Encoder 14bit v5 (Autodesk Fusion 360 design; units mm, degrees)
Autodesk Fusion 360 part; units mm, degrees
sketch "Sketch1" plane through (0, 0, 0) normal (0, 0, 1) x (1, 0, 0)
  circle A0 centre (-8.5, 8.5) radius 1
  line L0 (-10.5, 11.5) -> (10.5, 11.5)
  line L1 (11.5, 10.5) -> (11.5, -10.5)
  line L2 (10.5, -11.5) -> (-10.5, -11.5)
  line L3 (-11.5, -10.5) -> (-11.5, 10.5)
  line L4 (-9.5, 11.5) -> (-9.5, 8.5) construction
  line L5 (-7.5, 11.5) -> (-7.5, 8.5) construction
  line L6 (-8.5, 9.5) -> (-11.5, 9.5) construction
  line L7 (0, 11.5) -> (0, -11.5) construction
  line L8 (-11.5, 0) -> (11.5, 0) construction
  circle A1 centre (8.5, 8.5) radius 1
  circle A2 centre (8.5, -8.5) radius 1
  circle A3 centre (-8.5, -8.5) radius 1
  line L9 (-10.5, 11.5) -> (-11.5, 10.5)
  line L10 (10.5, 11.5) -> (11.5, 10.5)
  line L11 (11.5, -10.5) -> (10.5, -11.5)
  line L12 (-10.5, -11.5) -> (-11.5, -10.5)
  point P0 (-11.5, 11.5)
  point P1 (11.5, 11.5)
  point P2 (11.5, -11.5)
  point P3 (-11.5, -11.5)
  dimension "d2" = 23
  dimension "d3" = 23
  dimension "d5" = 2
  dimension "d6" = 19
  dimension "d7" = 2
  dimension "d8" = 1
  dimension "d9" = 1
  dimension "d10" = 1
  dimension "d11" = 1
  dimension "d12" = 1
  dimension "d13" = 1
  dimension "d14" = 1
  dimension "d15" = 1
  constraint horizontal L0
  constraint vertical L1
  constraint horizontal L2
  constraint vertical L3
  constraint coincident L0 L4.start
  constraint perpendicular L0 L4
  constraint coincident L0 L5.start
  constraint perpendicular L0 L5
  constraint tangent A0 L4
  constraint tangent A0 L5
  constraint coincident A0 L4.end
  constraint coincident A0 L5.end
  constraint coincident A0 L6.start
  constraint coincident L3 L6.end
  constraint tangent A0 L6
  constraint perpendicular L3 L6
  constraint symmetric A0 L7 A1
  constraint symmetric A0 L8 A3
  constraint symmetric L8 A1 A2
  constraint midpoint L7 origin
  constraint coincident L0 L7.start
  constraint coincident L3 L8.start
  constraint coincident P0 L0
  constraint coincident P0 L3
  constraint coincident L1 L8.end
  constraint coincident P1 L0
  constraint coincident P1 L1
  constraint coincident L2 L7.end
  constraint coincident P2 L1
  constraint coincident P2 L2
  constraint coincident P3 L2
  constraint coincident P3 L3
  measures "d2" distance of P0 P1
  measures "d3" distance of P0 P3
  measures "d5" distance of L3 L4
  measures "d6" distance of L1 L5
  measures "d7" distance of L0 L6
  measures "d8" distance of P0 L0.start
  measures "d9" distance of P0 L3.end
  measures "d10" distance of P1 L0.end
  measures "d11" distance of P1 L1.start
  measures "d12" distance of P2 L1.end
  measures "d13" distance of P2 L2.start
  measures "d14" distance of P3 L2.end
  measures "d15" distance of P3 L3.start
extrude "Extrude1" add sketch "Sketch1" along normal blind 1.6
sketch "Sketch2" plane through (0, 0, 1.6) normal (0, 0, 1) x (-1, 0, 0)
  circle A0 centre (8.5, 8.5) radius 1
  circle A1 centre (-8.5, -8.5) radius 1
  circle A2 centre (-8.5, 8.5) radius 1
  circle A3 centre (8.5, -8.5) radius 1
  line L0 (10.5, -11.5) -> (11.5, -10.5)
  line L1 (11.5, -10.5) -> (11.5, 10.5)
  line L2 (11.5, 10.5) -> (10.5, 11.5)
  line L3 (10.5, 11.5) -> (-10.5, 11.5)
  line L4 (-10.5, 11.5) -> (-11.5, 10.5)
  line L5 (-11.5, 10.5) -> (-11.5, -10.5)
  line L6 (-11.5, -10.5) -> (-10.5, -11.5)
  line L7 (-10.5, -11.5) -> (10.5, -11.5)
  line L8 (1.9, -2.6) -> (-1.9, -2.6)
  line L9 (-1.9, -2.6) -> (-1.9, 2.6)
  line L10 (-1.9, 2.6) -> (1.9, 2.6)
  line L11 (1.9, 2.6) -> (1.9, -2.6)
  line L12 (11, -11) -> (-11, 11) construction
  line L13 (-11, -11) -> (11, 11) construction
  line L14 (1.9, -2.6) -> (-1.9, 2.6) construction
  line L15 (1.9, 2.6) -> (-1.9, -2.6) construction
  line L16 (6.75, 6.8) -> (-6.75, 6.8)
  line L17 (6.75, 5.3) -> (-6.75, 5.3)
  line L18 (-6.75, 5.3) -> (-6.75, 8.3)
  line L19 (-6.75, 8.3) -> (6.75, 8.3)
  line L20 (6.75, 8.3) -> (6.75, 5.3)
  line L21 (0, 6.8) -> (0, 11.5) construction
  dimension "d18" = 5.2
  dimension "d19" = 3.8
  dimension "d23" = 4.7
  dimension "d24" = 3
  dimension "d25" = 13.5
  constraint horizontal L8
  constraint vertical L9
  constraint horizontal L10
  constraint vertical L11
  constraint midpoint L0 L12.start
  constraint midpoint L4 L12.end
  constraint midpoint L6 L13.start
  constraint midpoint L2 L13.end
  constraint midpoint L14 origin
  constraint horizontal L16
  constraint horizontal L17
  constraint vertical L18
  constraint horizontal L19
  constraint vertical L20
  constraint coincident L16.end L18
  constraint midpoint L16.start L20
  constraint midpoint L16 L21.start
  constraint coincident L3 L21.end
  constraint perpendicular L3 L21
  constraint midpoint L3 L21.end
  measures "d18" distance of L8.end L9.end
  measures "d19" distance of L8.start L8.end
  measures "d23" distance of L3 L16
  measures "d24" distance of L17.start L19.end
  measures "d25" distance of L17.start L17.end
extrude "Extrude2" add sketch "Sketch2" along normal blind 1.8 contours L8 L9 L10 L11
chamfer "Chamfer1" distance 0.4 angle 45 1 faces at (-0.6333, 0.8667, 3.4)
extrude "Extrude3" add sketch "Sketch2" along normal blind 1.5 contours L16 L17 L18 L20 | L16 L18 L19 L20
sketch "Sketch3" plane through (0, 0, 3.4) normal (0, 0, 1) x (-1, 0, 0)
  line L0 (-1.5, -2.2) -> (1.5, -2.2)
  line L1 (1.5, -2.2) -> (1.5, 2.2)
  line L2 (1.5, 2.2) -> (-1.5, 2.2)
  line L3 (-1.5, 2.2) -> (-1.5, -2.2)
equation "d7 = d5"
equation "d9 = d8"
equation "d11 = d10"
equation "d13 = d12"
equation "d15 = d14"
